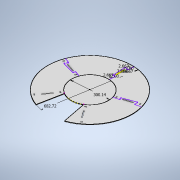
# Autodesk Inventor part: Ring D Full
Saved by Autodesk Inventor 2020 (Build 240168000, 168)
## iProperties
Created: 2020-03-10
Part Number: Ring D Full
Material: Generic
Document SubType Name: Sheet Metal
Designer: Daniel Wikman
Density: 1 g/cm^3
Sheet Metal Rule: Default_mm
Appearance: Default
Author: Daniel Wikman
Autodesk Inventor part; units mm, degrees
ref_plane "YZ Plane" through (0, 0, 0) normal (1, 0, 0) x (0, 1, 0)
ref_plane "XZ Plane" through (0, 0, 0) normal (0, 1, 0) x (-1, 0, 0)
ref_plane "XY Plane" through (0, 0, 0) normal (0, 0, 1) x (1, 0, 0)
sketch "Sketch1" plane through (0, 0, 0) normal (0, 1, 0) x (-1, 0, 0)
  circle A0 centre (0, 0) radius 341.36
  circle A1 centre (0, 0) radius 150.07
  dimension "d84" = 300.14
  dimension "d85" = 682.72
  constraints: 2 centre point, 1 coincident
  measures "d84" diameter of A1
  measures "d85" diameter of A0
extrude "Extrusion3" add sketch "Sketch1" along normal blind 6 contours A0 | A1
sketch "Sketch2" plane through (0, 6, 0) normal (0, 1, 0) x (1, 0, 0)
  circle A0 centre (0, 0) radius 245.715 construction
  line L0 (245.7148, 0.3131) -> (341.6521, -0.0088)
  line L1 (3.25, 279.0483) -> (3.25, 212.3817)
  line L2 (-3.25, 212.3817) -> (-3.25, 279.0483)
  arc A1 (-3.25, 212.3817) -> (-1.9167, 211.0483) centre (-1.9167, 212.3817) ccw
  arc A2 (1.9167, 211.0483) -> (3.25, 212.3817) centre (1.9167, 212.3817) ccw
  arc A3 (-1.9167, 280.3817) -> (-3.25, 279.0483) centre (-1.9167, 279.0483) ccw
  arc A4 (3.25, 279.0483) -> (1.9167, 280.3817) centre (1.9167, 279.0483) ccw
  line L3 (-1.9167, 280.3817) -> (1.9167, 280.3817)
  line L4 (-1.9167, 211.0483) -> (1.9167, 211.0483)
  line L5 (0, 0) -> (0, 212.3817)
  line L6 (0, 280.3817) -> (0, 341.36)
  line L7 (0, 211.0483) -> (0, 245.715) construction
  line L8 (0, 280.3817) -> (0, 245.715) construction
  line L9 (-266.6835, 86.5666) -> (-233.7136, 75.854) construction
  line L10 (-264.4112, 89.2455) -> (-201.0074, 68.6444)
  arc A5 (-200.1513, 66.9643) -> (-201.0074, 68.6444) centre (-201.4194, 67.3763) ccw
  line L11 (-200.7436, 65.1414) -> (-233.7136, 75.854) construction
  line L12 (-201.3359, 63.3186) -> (-200.1513, 66.9643)
  line L13 (-267.2758, 84.7438) -> (-266.0912, 88.3895)
  line L14 (-203.016, 62.4625) -> (-266.4198, 83.0637)
  arc A6 (-203.016, 62.4625) -> (-201.3359, 63.3186) centre (-202.604, 63.7306) ccw
  arc A7 (-267.2758, 84.7438) -> (-266.4198, 83.0637) centre (-266.0077, 84.3317) ccw
  arc A8 (-264.4112, 89.2455) -> (-266.0912, 88.3895) centre (-264.8232, 87.9775) ccw
  line L15 (-165.0631, -226.6454) -> (-144.6865, -198.5995) construction
  line L16 (-166.9087, -223.6565) -> (-127.723, -169.722)
  arc A9 (-125.8606, -169.427) -> (-127.723, -169.722) centre (-126.6443, -170.5057) ccw
  line L17 (-124.31, -170.5536) -> (-144.6865, -198.5995) construction
  line L18 (-122.7594, -171.6802) -> (-125.8606, -169.427)
  line L19 (-163.5125, -227.772) -> (-166.6137, -225.5189)
  line L20 (-122.4644, -173.5426) -> (-161.6501, -227.4771)
  arc A10 (-122.4644, -173.5426) -> (-122.7594, -171.6802) centre (-123.5431, -172.7589) ccw
  arc A11 (-163.5125, -227.772) -> (-161.6501, -227.4771) centre (-162.7288, -226.6933) ccw
  arc A12 (-166.9087, -223.6565) -> (-166.6137, -225.5189) centre (-165.83, -224.4402) ccw
  line L21 (164.8042, -226.8335) -> (144.4277, -198.7876) construction
  line L22 (160.9139, -228.0119) -> (121.7282, -174.0775)
  arc A13 (122.0232, -172.2151) -> (121.7282, -174.0775) centre (122.8069, -173.2938) ccw
  line L23 (123.5738, -171.0885) -> (144.4277, -198.7876) construction
  line L24 (125.1244, -169.9619) -> (122.0232, -172.2151)
  line L25 (165.8775, -226.0537) -> (162.7763, -228.3069)
  line L26 (126.9868, -170.2569) -> (166.1725, -224.1913)
  arc A14 (126.9868, -170.2569) -> (125.1244, -169.9619) centre (125.9081, -171.0406) ccw
  arc A15 (165.8775, -226.0537) -> (166.1725, -224.1913) centre (165.0938, -224.975) ccw
  arc A16 (160.9139, -228.0119) -> (162.7763, -228.3069) centre (161.9926, -227.2282) ccw
  line L27 (266.7793, 86.2718) -> (233.8094, 75.5592) construction
  line L28 (266.5156, 82.7688) -> (203.1118, 62.1677)
  arc A17 (201.4317, 63.0238) -> (203.1118, 62.1677) centre (202.6998, 63.4358) ccw
  line L29 (200.8394, 64.8466) -> (233.8094, 75.5592) construction
  line L30 (200.2471, 66.6695) -> (201.4317, 63.0238)
  line L31 (266.187, 88.0946) -> (267.3716, 84.4489)
  line L32 (201.1032, 68.3496) -> (264.5069, 88.9507)
  arc A18 (201.1032, 68.3496) -> (200.2471, 66.6695) centre (201.5152, 67.0815) ccw
  arc A19 (266.187, 88.0946) -> (264.5069, 88.9507) centre (264.919, 87.6826) ccw
  arc A20 (266.5156, 82.7688) -> (267.3716, 84.4489) centre (266.1035, 84.0369) ccw
  point P0 (-202.0117, 65.5535)
  point P1 (-125.0937, -171.6323)
  point P2 (124.8348, -171.8204)
  point P3 (202.1075, 65.2586)
  dimension "d21" = 6.5
  dimension "d24" = 2.6667
  dimension "d25" = 2.6667
  dimension "d32" = 1.3333
  dimension "d33" = 1.3333
  dimension "d41" = 90
  dimension "d42" = 3.25
  dimension "d43" = 90
  dimension "d86" = 491.43
  constraints: 66 end point, 42 point on circle, 21 centre point, 8 midpoint, 6 tangent, 2 equal length, 2 point on line, 2 vertical, 1 coincident, 1 collinear
  measures "d21" distance between parallel lines of L1 L2
  measures "d24" diameter of A1
  measures "d25" diameter of A2
  measures "d32" radius of A3
  measures "d33" radius of A4
  measures "d41" angle of L4 L5
  measures "d42" distance between parallel lines of L5 L1
  measures "d43" angle of L3 L6
  measures "d86" diameter of A0
extrude "Extrusion4" cut sketch "Sketch2" against normal through all
sketch "Sketch3" plane through (0, 6, 0) normal (0, 1, 0) x (1, 0, 0)
  arc A0 (-115.2299, -321.3234) -> (115.2355, -321.3214) centre (0, 0) ccw
  arc A1 (-77.7244, -128.3741) -> (77.7297, -128.3709) centre (0, 0) ccw
  line L0 (-122.1811, -173.696) -> (-161.3589, -227.6196)
  line L1 (-115.2299, -321.3234) -> (-77.7244, -128.3741)
  line L2 (0, 0) -> (0, -341.2918)
  line L3 (115.2355, -321.3214) -> (77.7297, -128.3709)
  line L4 (161.3912, -227.6651) -> (122.2055, -173.7307) projected
  dimension "d52" = 25
  dimension "d87" = 150.07
  dimension "d88" = 341.36
  dimension "d89" = 25
  dimension "d90" = 11
  dimension "d91" = 11
  constraints: 8 end point, 4 point on circle, 2 centre point, 1 coincident
  measures "d52" angle of L0 L1
  measures "d87" radius of A1
  measures "d88" radius of A0
  measures "d89" angle of L4 L3
  measures "d90" angle of L3 L2
  measures "d91" angle of L1 L2
extrude "Extrusion5" cut sketch "Sketch3" against normal blind 10
sketch "Sketch5" plane through (0, 6, 0) normal (0, 1, 0) x (1, 0, 0)
  line L0 (3.25, 279.0483) -> (3.25, 212.3817) projected
  line L1 (5.5862, 197.9634) -> (-6.155, 194.8174)
  line L2 (-11.2263, 301.7146) -> (10.5847, 293.3421)
  line L3 (6.5657, 149.9554) -> (8.9394, 195.248)
  line L4 (14.2034, 295.6921) -> (16.5771, 340.9846)
  arc A0 (10.5847, 293.3421) -> (14.2034, 295.6921) centre (11.5404, 295.8316) ccw
  arc A1 (8.9394, 195.248) -> (5.5862, 197.9634) centre (6.2763, 195.3876) ccw
  arc A2 (-11.2263, 301.7146) -> (-14.8449, 299.0854) centre (-12.1819, 299.225) ccw
  line L5 (-3.25, 212.3817) -> (-3.25, 279.0483) projected
  line L6 (-14.8449, 299.0854) -> (-9.5081, 197.2536)
  arc A3 (-9.5081, 197.2536) -> (-6.155, 194.8174) centre (-6.8451, 197.3932) ccw
  line L7 (-1.9167, 211.0483) -> (1.9167, 211.0483) projected
  line L8 (1.9167, 280.3817) -> (-1.9167, 280.3817) projected
  arc A4 (115.2355, -321.3214) -> (-115.2299, -321.3234) centre (0, 0) ccw
  line L9 (16.5771, 340.9846) -> (16.5774, 340.9903)
  arc A5 (-190.5375, 51.9119) -> (-187.1843, 54.3482) centre (-189.8473, 54.4877) ccw
  line L10 (-186.5481, 66.4868) -> (-187.1843, 54.3482)
  arc A6 (-182.9295, 68.8368) -> (-186.5481, 66.4868) centre (-183.8851, 66.3472) ccw
  arc A7 (-275.714, 100.7144) -> (-276.8308, 104.8821) centre (-277.7864, 102.3926) ccw
  line L11 (-289.0345, 78.3041) -> (-190.5375, 51.9119)
  arc A8 (-290.4167, 82.5581) -> (-289.0345, 78.3041) centre (-288.3443, 80.8799) ccw
  line L12 (-290.4167, 82.5581) -> (-275.714, 100.7144)
  line L13 (-276.8308, 104.8821) -> (-319.1731, 121.1358)
  line L14 (-140.5872, 52.5831) -> (-182.9295, 68.8368)
  line L15 (-319.1731, 121.1358) -> (-319.1784, 121.1378)
  arc A9 (184.6611, 69.9975) -> (183.3803, 66.0556) centre (185.6168, 67.508) ccw
  line L16 (190.0006, 55.8613) -> (183.3803, 66.0556)
  arc A10 (188.4543, 51.8331) -> (190.0006, 55.8613) centre (187.7641, 54.4089) ccw
  arc A11 (282.2558, 80.581) -> (285.609, 77.8656) centre (284.9188, 80.4414) ccw
  line L17 (279.8598, 106.5409) -> (184.6611, 69.9975)
  arc A12 (283.4785, 103.9117) -> (279.8598, 106.5409) centre (280.8155, 104.0513) ccw
  line L18 (283.4785, 103.9117) -> (282.2558, 80.581)
  line L19 (285.609, 77.8656) -> (329.4183, 89.6043)
  line L20 (144.645, 40.0945) -> (188.4543, 51.8331)
  line L21 (329.4183, 89.6043) -> (329.4238, 89.6058)
  circle A13 centre (0, 0) radius 150.07
  line L22 (-140.5872, 52.5831) -> (-140.5479, 52.568)
  line L23 (144.645, 40.0945) -> (144.5122, 40.0589)
  line L24 (6.5657, 149.9554) -> (6.5621, 149.8874)
  arc A14 (-77.7244, -128.3741) -> (77.7297, -128.3709) centre (0, 0) ccw projected
  arc A15 (115.2355, -321.3214) -> (-115.2299, -321.3234) centre (0, 0) ccw projected
  line L25 (77.7297, -128.3709) -> (115.2355, -321.3214)
  line L26 (-77.7244, -128.3741) -> (-115.2299, -321.3234)
  point P0 (-77.7399, -128.3998)
  point P1 (77.7399, -128.3998)
  point P2 (-319.1475, 121.126)
  point P3 (-140.56, 52.5727)
  point P4 (6.5642, 149.9264)
  point P5 (16.5757, 340.9573)
  point P6 (329.3918, 89.5972)
  point P7 (144.6169, 40.0869)
  dimension "d63" = 2.6667
  dimension "d64" = 3
  dimension "d66" = 3
  dimension "d67" = 2.6667
  dimension "d68" = 2.6667
  dimension "d70" = 72
  dimension "d71" = 72
  dimension "d94" = 300.14
  dimension "d95" = 682.72
  constraints: 46 end point, 26 point on circle, 14 centre point, 8 tangent, 2 collinear, 1 coincident, 1 equal radius
  measures "d63" radius of A0
  measures "d64" angle of L0 L4
  measures "d66" angle of L5 L6
  measures "d67" radius of A2
  measures "d68" radius of A3
  measures "d70" angle of L3 L1
  measures "d71" angle of L4 L2
  measures "d94" diameter of A13
  measures "d95" diameter of A4
sketch "Sketch6" plane through (0, 6, 0) normal (0, 1, 0) x (1, 0, 0)
  line L0 (188.7727, -264.2184) -> (198.4809, -257.165)
  line L1 (194.6603, -251.9064) -> (184.9521, -258.9598)
  line L2 (161.3912, -227.6651) -> (122.2055, -173.7307) projected
  line L3 (166.3548, -225.7069) -> (163.2536, -227.9601) projected
  arc A0 (195.5915, -252.0539) -> (194.6603, -251.9064) centre (195.0522, -252.4457) ccw
  arc A1 (198.4809, -257.165) -> (198.6284, -256.2338) centre (198.0891, -256.6256) ccw
  arc A2 (187.8415, -264.0709) -> (188.7727, -264.2184) centre (188.3809, -263.6791) ccw
  arc A3 (184.9521, -258.9598) -> (184.8046, -259.891) centre (185.344, -259.4991) ccw
  line L4 (184.8046, -259.891) -> (187.8415, -264.0709)
  line L5 (198.6284, -256.2338) -> (195.5915, -252.0539)
  line L6 (122.2055, -173.7307) -> (161.3912, -227.6651) projected
  line L7 (141.7983, -200.6979) -> (147.057, -196.8773)
  line L8 (166.6498, -223.8445) -> (127.4641, -169.9101) projected
  line L9 (95.9027, -136.3937) -> (105.6109, -129.3403)
  line L10 (109.4315, -134.5989) -> (99.7233, -141.6523)
  arc A4 (109.4315, -134.5989) -> (109.579, -133.6677) centre (109.0396, -134.0596) ccw
  arc A5 (106.5421, -129.4878) -> (105.6109, -129.3403) centre (106.0027, -129.8796) ccw
  arc A6 (95.9027, -136.3937) -> (95.7552, -137.3249) centre (96.2945, -136.9331) ccw
  arc A7 (98.7921, -141.5048) -> (99.7233, -141.6523) centre (99.3314, -141.113) ccw
  line L11 (98.7921, -141.5048) -> (95.7552, -137.3249)
  line L12 (106.5421, -129.4878) -> (109.579, -133.6677)
  point P0 (0, 0)
  dimension "d104" = 6.5
  dimension "d105" = 12
  dimension "d108" = 1.3333
  dimension "d109" = 1.3333
  dimension "d110" = 1.3333
  dimension "d111" = 1.3333
  dimension "d112" = 0
  dimension "d149" = 145
  dimension "d150" = 90
  dimension "d151" = 90
  dimension "d152" = 90
  dimension "d153" = 90
  constraints: 18 end point, 16 point on circle, 12 symmetric about line, 8 centre point, 8 tangent, 2 midpoint, 4 other
  measures "d104" distance of L1.end L0.start
  measures "d105" distance of L0.start L0.end
  measures "d108" diameter of A0
  measures "d109" diameter of A1
  measures "d110" diameter of A2
  measures "d111" diameter of A3
  measures "d112" distance between parallel lines of L2 L4
  measures "d149" diameter of L1 L7
  measures "d150" angle of L5 L1
  measures "d151" angle of L0 L5
  measures "d152" angle of L4 L0
  measures "d153" angle of L1 L4
extrude "Extrusion7" cut sketch "Sketch6" against normal through all
pattern_circular "Circular Pattern2" count 2 over 72 about axis through (0, -10, 0) along (0, 1, 0) of "Extrusion7"
pattern_circular "Circular Pattern3" count 2 over 144 about axis through (0, -10, 0) along (0, 1, 0) of "Extrusion7"
mirror "Mirror3" about plane through (0, 0, 0) normal (1, 0, 0) of "Extrusion7"
pattern_circular "Circular Pattern4" count 2 over 144 about axis through (0, -10, 0) along (0, -1, 0) of "Extrusion7"
equation "\"BendRadius\" = Thickness"
equation "\"BendReliefWidth\" = Thickness"
equation "\"BendReliefDepth\" = 0.5 * Thickness"
equation "\"CornerReliefSize\" = 4 * Thickness"
equation "\"MinimumRemnant\" = 2 * Thickness"
equation "\"TransitionRadius\" = BendRadius"
equation "\"JacobiRadiusSize\" = BendRadius"
equation "\"GapSize\" = Thickness"
equation "\"Thickness\" = 0.5"
body "Solid3"
